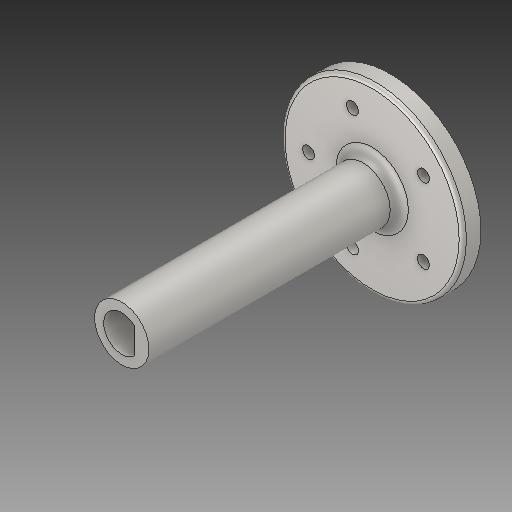
# Autodesk Inventor part: 342-01
Saved by Autodesk Inventor 2019 (Build 230136000, 136)
## iProperties
Company: Autodesk Inc.
Created: 2017-06-23
Part Number: 342-01
Material: Titanium
Document SubType Name: Modeling
Designer: Autodesk Inc.
Density: 4.51 g/cm^3
Appearance: Stainless - Brushed
Mass: 592.694 g
Surface Area: 404.589 cm^2
Volume: 131.418 cm^3
Author: Inventor
Autodesk Inventor part; units mm, degrees
ref_plane "YZ Plane" through (0, 0, 0) normal (1, 0, 0) x (0, 1, 0)
ref_plane "XZ Plane" through (0, 0, 0) normal (0, 1, 0) x (-1, 0, 0)
ref_plane "XY Plane" through (0, 0, 0) normal (0, 0, 1) x (1, 0, 0)
sketch "Sketch2" plane through (0, 0, 0) normal (0, 0, 1) x (1, 0, 0)
  circle A0 centre (0, 0) radius 50
  arc A1 (7.1414, 7) -> (7.1414, -7) centre (0, 0) ccw
  line L0 (7.1414, -7) -> (7.1414, 7)
  dimension "d2" = 100
  dimension "d3" = 20
  dimension "d23" = 14
  constraints: 2 centre point, 2 coincident, 2 end point, 2 point on circle, 1 vertical
  measures "d2" diameter of A0
  measures "d3" diameter of A1
  measures "d23" distance of L0.start L0.end
extrude "Extrusion1" add sketch "Sketch2" along normal blind 10
sketch "Sketch3" plane through (0, 0, 10) normal (0, 0, 1) x (1, 0, 0)
  circle A0 centre (0, 0) radius 15
  line L0 (7.1414, 7) -> (7.1414, -7) projected
  arc A1 (7.1414, 7) -> (7.1414, -7) centre (0, 0) ccw projected
  circle A2 centre (0, 0) radius 50 projected
  dimension "d6" = 30
  constraints: 1 centre point, 1 coincident
  measures "d6" diameter of A0
extrude "Extrusion2" add sketch "Sketch3" along normal blind 138 contours A0
fillet "Fillet1" radius 2 1 edges at (-50, 0, 10)
fillet "Fillet2" radius 5 1 edges at (-15, 0, 10)
sketch "Sketch4" plane through (0, 0, 0) normal (0, 0, -1) x (-1, 0, 0)
  circle A0 centre (35, 0) radius 6
  point P0 (0, 0)
  dimension "d11" = 35
  dimension "d12" = 12
  constraints: 1 centre point
  measures "d11" distance of A0.centre point (0, 0)
  measures "d12" diameter of A0
hole "Hole1" at (-35, 0, 0) direction (0, 0, 1) diameter 6.6 end through all countersink diameter 13.44 countersink angle 90
pattern_circular "Circular Pattern1" count 5 over 360 about axis through (0, 0, 0) along (0, 0, 1) of "Hole1"
body "Solid1"
